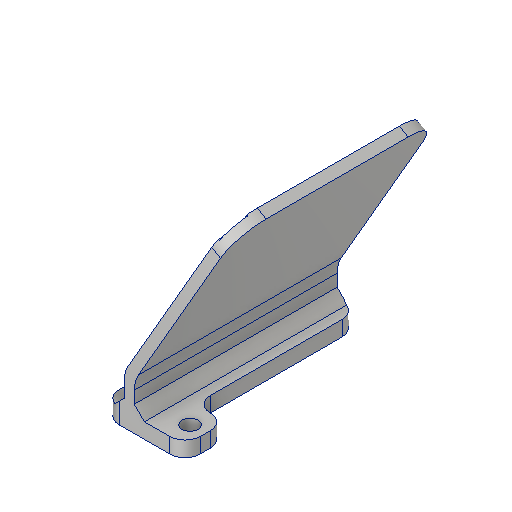
# Autodesk Inventor part: CNCM_ALU_Camera_calibration_marker
Saved by Autodesk Inventor 2025 (Build 290162010, 162A)
## iProperties
Created: 2018-09-21
Part Number: CNCM_ALU_Camera_calibration_marker
Material: Aluminum 6061
Document SubType Name: Modeling
Designer: Andrzej
Density: 2.7 g/cm^3
Appearance: Aluminum - Flat
Author: Andrzej
Autodesk Inventor part; units mm, degrees
ref_plane "YZ Plane" through (0, 0, 0) normal (1, 0, 0) x (0, 1, 0)
ref_plane "XZ Plane" through (0, 0, 0) normal (0, 1, 0) x (-1, 0, 0)
ref_plane "XY Plane" through (0, 0, 0) normal (0, 0, 1) x (1, 0, 0)
sketch "Sketch1" plane through (0, 0, 0) normal (0, 0, 1) x (1, 0, 0)
  line L0 (0, 0) -> (0, 3)
  line L1 (0, 3) -> (10, 20.3205)
  line L2 (10, 20.3205) -> (9.134, 20.8205)
  line L3 (9.134, 20.8205) -> (-1, 3.2679)
  line L4 (-1, 3.2679) -> (-1, 0)
  line L5 (-1, 0) -> (-3, 0)
  line L6 (-3, 0) -> (-3, -1.5)
  line L7 (-3, -1.5) -> (2, -1.5)
  line L8 (2, -1.5) -> (2, 0)
  line L9 (2, 0) -> (0, 0)
  dimension "d0" = 3
  dimension "d1" = 20
  dimension "d2" = 150
  dimension "d3" = 1
  dimension "d4" = 1.5
  dimension "d5" = 2
  dimension "d6" = 2
  dimension "d10" = 1
  constraints: 20 end point, 5 perpendicular, 2 vertical, 1 horizontal, 1 point on line
  measures "d0" distance of L0.start L0.end
  measures "d1" distance of L0.end L1.end
  measures "d2" angle of L0 L1
  measures "d3" distance of L1.end L2.end
  measures "d4" distance of L5.end L6.end
  measures "d5" distance of L4.end L5.end
  measures "d6" distance of L8.end L0.start
  measures "d10" distance between parallel lines of L4 L0
extrude "Extrusion1" add sketch "Sketch1" along normal blind 20
sketch "Sketch2" plane through (-1, 3.2679, 0) normal (-0.8660254, 0.5, 0) x (0, 0, 1)
  line L0 (0, 20.2679) -> (0, 0) projected
  line L1 (0, 0) -> (20, 0) projected
  line L2 (20, 20.2679) -> (20, 0) projected
  line L3 (0, 20.2679) -> (20, 20.2679) projected
  circle A0 centre (10, 10.134) radius 5
  circle A1 centre (10, 10.134) radius 7.5
  circle A2 centre (10, 10.134) radius 8.75
  line L4 (0, 0.2679) -> (0, 20.2679) projected
  line L5 (0, 10.134) -> (1.25, 10.134)
  line L6 (2.5, 10.134) -> (1.25, 10.134)
  line L7 (2.5, 10.134) -> (5, 10.134)
  line L8 (5, 10.134) -> (15, 10.134)
  line L9 (15, 10.134) -> (17.5, 10.134)
  line L10 (17.5, 10.134) -> (18.75, 10.134)
  line L11 (18.75, 10.134) -> (20, 10.134)
  line L12 (0, 0) -> (20, 0) projected
  line L13 (10, 0) -> (10, 1.384)
  line L14 (10, 2.634) -> (10, 1.384)
  line L15 (10, 2.634) -> (10, 5.134)
  line L16 (10, 5.134) -> (10, 10.134)
  line L17 (10, 10.134) -> (10, 15.134)
  line L18 (10, 15.134) -> (10, 17.634)
  line L19 (10, 17.634) -> (10, 18.884)
  line L20 (10, 20.2679) -> (10, 18.884)
  line L21 (16.8937, 2.799) -> (18.8937, 2.799)
  line L22 (18.8937, 2.799) -> (18.8937, 0.799)
  line L23 (18.8937, 0.799) -> (16.8937, 0.799)
  line L24 (16.8937, 0.799) -> (16.8937, 2.799)
  line L25 (18, 20.2679) -> (17.6063, 17.8743)
  line L26 (17.6063, 17.8743) -> (20, 18.2679)
  line L27 (20, 0.2679) -> (20, 20.2679) projected
  circle A3 centre (1.875, 18.2679) radius 1
  circle A4 centre (1.875, 1.799) radius 1.5
  dimension "d19" = 10
  dimension "d20" = 15
  dimension "d21" = 17.5
  dimension "d22" = 2
  dimension "d23" = 2
  dimension "d24" = 2
  dimension "d25" = 2
  dimension "d26" = 2.3937
  dimension "d27" = 2.3937
  dimension "d28" = 2
  dimension "d29" = 3
  constraints: 42 end point, 13 point on circle, 13 point on line, 5 centre point, 3 midpoint, 3 perpendicular, 2 coincident, 2 collinear, 2 parallel, 1 horizontal, 1 vertical
  measures "d19" diameter of A0
  measures "d20" diameter of A1
  measures "d21" diameter of A2
  measures "d22" distance of L22.end L23.end
  measures "d23" distance of L21.end L22.end
  measures "d24" distance of L2.start L25.start
  measures "d25" distance of L2.start L26.end
  measures "d26" horizontal distance of L25.end L26.end
  measures "d27" distance from line of L3 L25.end
  measures "d28" diameter of A3
  measures "d29" diameter of A4
extrude "Extrusion3" cut sketch "Sketch2" against normal blind 0.1 contours A2 L19 A1 L6 | L3 L2 L26 L25 | L14 A1 L10 A2 | L7 A0 L15 A1 | A1 L9 A0 L18 | L21 L22 L23 L24 | A3 | A4
sketch "Sketch3" plane through (4.067, 12.0442, 2.5) normal (-0.8660254, 0.5, 0) x (0, 0, 1)
  arc A0 (7.5, 7.5) -> (0, 0) centre (7.5, 0) ccw projected
  line L0 (0, 0) -> (2.5, 0) projected
  arc A1 (2.5, 0) -> (7.5, -5) centre (7.5, 0) ccw projected
  line L1 (7.5, -5) -> (7.5, -7.5) projected
  arc A2 (7.5, -7.5) -> (15, 0) centre (7.5, 0) ccw projected
  line L2 (15, 0) -> (12.5, 0) projected
  arc A3 (12.5, 0) -> (7.5, 5) centre (7.5, 0) ccw projected
  line L3 (7.5, 5) -> (7.5, 7.5) projected
  arc A4 (12.5, 0) -> (7.5, 5) centre (7.5, 0) ccw projected
  circle A5 centre (7.5, 0) radius 5
  line L4 (2.5, 0) -> (7.5, 0)
  line L5 (7.5, 0) -> (7.5, 5)
  line L6 (7.5, 0) -> (7.5, -5)
  line L7 (7.5, 0) -> (12.5, 0)
  point P0 (-2.5, -12.4641)
  constraints: 8 end point, 1 coincident, 1 collinear, 1 horizontal, 1 perpendicular, 1 vertical, 1 vertical alignment, 2 other
extrude "Extrusion4" cut sketch "Sketch3" against normal blind 0.1 contours L5 L4 A5 | A5 L6 L7
fillet "Fillet1" radius 3 2 edges at (9.567, 20.5705, 0) (9.6112, 20.545, 20)
chamfer "Chamfer1" distance 1 angle 45 2 edges at (-1, 0, 10) (0, 0, 10)
fillet "Fillet2" radius 3 2 edges at (0, 3, 10) (-1, 3.2679, 10)
sketch "Sketch4" plane through (-3, -1.5, 0) normal (-1, 0, 0) x (0, 0, 1)
  line L0 (0, 0) -> (0, 1.5) projected
  line L1 (20, 1.5) -> (0, 1.5) projected
  line L2 (0, 0) -> (4, 0)
  line L3 (4, 0) -> (4, 1.5)
  line L4 (4, 1.5) -> (0, 1.5)
  line L5 (0, 1.5) -> (0, 0)
  dimension "d39" = 4
  constraints: 8 end point, 2 parallel, 1 horizontal, 1 perpendicular, 1 point on line
  measures "d39" distance of L4.end L3.end
extrude "Extrusion5" add sketch "Sketch4" along normal blind 3
sketch "Sketch5" plane through (2, -1.5, 0) normal (1, 0, 0) x (0, 0, -1)
  line L0 (0, 0) -> (0, 1.5) projected
  line L1 (0, 1.5) -> (-20, 1.5) projected
  line L2 (-20, 0) -> (-20, 1.5) projected
  line L3 (0, 0) -> (-20, 0) projected
  line L4 (0, 0) -> (-20, 0) projected
  line L5 (-20, 1.5) -> (0, 1.5) projected
  line L6 (-20, 0) -> (-16, 0)
  line L7 (-16, 0) -> (-16, 1.5)
  line L8 (-16, 1.5) -> (-20, 1.5)
  line L9 (-20, 1.5) -> (-20, 0)
  dimension "d42" = 4
  constraints: 8 end point, 2 parallel, 1 horizontal, 1 perpendicular, 1 point on line
  measures "d42" distance of L8.end L7.end
extrude "Extrusion6" add sketch "Sketch5" along normal blind 3 contours L3 L2 L1 L7
sketch "Sketch6" plane through (-6, -1.5, 0) normal (0, -1, 0) x (1, 0, 0)
  line L0 (8, 0) -> (0, 0) projected
  line L1 (8, 0) -> (8, 16) projected
  line L2 (8, 16) -> (11, 16) projected
  line L3 (11, 20) -> (11, 16) projected
  line L4 (3, 20) -> (11, 20) projected
  line L5 (3, 4) -> (3, 20) projected
  line L6 (3, 4) -> (0, 4) projected
  line L7 (0, 0) -> (0, 4) projected
  point P0 (6, 0)
  point P1 (9.5, 18)
  point P2 (1.5, 2)
hole "Hole1" at (3.5, -1.5, 18) at (-4.5, -1.5, 2) direction (0, 1, 0) diameter 1.6 depth 1.5 tip angle 118
fillet "Fillet3" radius 1.5 6 edges at (-3, -0.75, 4) (-6, -0.75, 4) (-6, -0.75, 0) (2, -0.75, 16) (5, -0.75, 16) (5, -0.75, 20)
fillet "Fillet3" radius 1.5 2 edges at (2, -0.75, 0) (-3, -0.75, 20)
equation "\"d6\" = d5"
equation "\"d10\" = d3"
equation "\"d25\" = d24"
equation "\"d27\" = d26"
body "Solid1"
